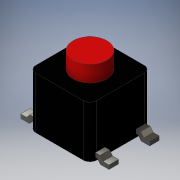
# Autodesk Inventor part: TL3305_Tactile
Saved by Autodesk Inventor 2016 (Build 200138000, 138)
## iProperties
Created: 2016-09-06
Part Number: TL3305_Tactile
Material: Generic
Document SubType Name: Modeling
Designer: jfixelle
Density: 1 g/cm^3
Appearance: Black
Author: jfixelle
Autodesk Inventor part; units mm, degrees
ref_plane "YZ Plane" through (0, 0, 0) normal (1, 0, 0) x (0, 1, 0)
ref_plane "XZ Plane" through (0, 0, 0) normal (0, 1, 0) x (-1, 0, 0)
sketch "Sketch1" plane through (0, 0, 0) normal (0, 1, 0) x (-1, 0, 0)
  line L0 (2.25, 2.25) -> (-2.25, 2.25)
  line L1 (-2.25, 2.25) -> (-2.25, -2.25)
  line L2 (-2.25, -2.25) -> (2.25, -2.25)
  line L3 (2.25, -2.25) -> (2.25, 2.25)
  point P0 (0, 0)
  dimension "d0" = 4.5
  dimension "d1" = 2.25
  dimension "d2" = 4.5
  dimension "d3" = 2.25
  constraints: 8 end point, 2 parallel, 1 horizontal, 1 perpendicular
  measures "d0" distance of L2.end L0.start
  measures "d1" distance from line of point (0, 0) L2
  measures "d2" distance of L1.end L2.end
  measures "d3" distance from line of point (0, 0) L3
extrude "Extrusion1" add sketch "Sketch1" along normal blind 3.8
fillet "Fillet1" radius 0.5 4 edges at (2.25, 1.9, 2.25) (2.25, 1.9, -2.25) (-2.25, 1.9, 2.25) (-2.25, 1.9, -2.25)
sketch "Sketch2" plane through (0, 3.8, 0) normal (0, 1, 0) x (1, 0, 0)
  circle A0 centre (0, 0) radius 1.25
  dimension "d7" = 2.5
  constraints: 1 centre point, 1 coincident
  measures "d7" diameter of A0
extrude "Extrusion2" add sketch "Sketch2" along normal blind 1.2
ref_plane "Work Plane1" through (0, 0, 1.5) normal (0, 0, 1) x (1, 0, 0)
sketch "Sketch3" plane through (0, 0, 1.5) normal (0, 0, 1) x (1, 0, 0)
  line L0 (-2.25, 3.8) -> (-2.25, 0) projected
  line L1 (-2.25, 0.5333) -> (-2.25, 0.2333)
  line L2 (-2.25, 0.2333) -> (-2.3946, 0.2333)
  line L3 (-2.3946, 0.2333) -> (-2.6231, -0.05)
  line L4 (-2.6231, -0.05) -> (-3.25, -0.05)
  line L5 (-3.25, -0.05) -> (-3.25, 0.25)
  line L6 (-3.25, 0.25) -> (-2.8162, 0.25)
  line L7 (-2.8162, 0.25) -> (-2.5878, 0.5333)
  line L8 (-2.5878, 0.5333) -> (-2.25, 0.5333)
  line L9 (-1.75, 0) -> (-2.25, 0) projected
  point P0 (0, 0)
  dimension "d11" = 0.3
  dimension "d12" = 0.3
  dimension "d13" = 0.05
  dimension "d14" = 1
  constraints: 16 end point, 3 parallel, 2 perpendicular, 2 point on line, 1 horizontal
  measures "d11" distance of L4.end L5.end
  measures "d12" distance between parallel lines of L2 L8
  measures "d13" distance between parallel lines of L9 L4
  measures "d14" distance between parallel lines of L5 L0
extrude "Extrusion3" add sketch "Sketch3" along normal mid plane 0.7
mirror "Mirror1" about plane through (0, 0, 0) normal (0, 0, 1) of "Extrusion3"
mirror "Mirror2" about plane through (0, 0, 0) normal (1, 0, 0) of "Extrusion3", "Mirror1"
body "Solid1"
